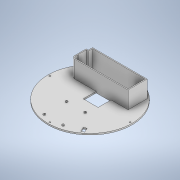
# Autodesk Inventor part: 07_CaseTop
Saved by Autodesk Inventor 2021 (Build 250183000, 183)
## iProperties
Created: 2021-06-07
Part Number: 07_CaseTop
Material: Generisch
Document SubType Name: Modeling
Designer: User
Density: 1 g/cm^3
Appearance: Vorgabe
Author: User
Autodesk Inventor part; units mm, degrees
ref_plane "YZ Plane" through (0, 0, 0) normal (1, 0, 0) x (0, 1, 0)
ref_plane "XZ Plane" through (0, 0, 0) normal (0, 1, 0) x (-1, 0, 0)
ref_plane "XY Plane" through (0, 0, 0) normal (0, 0, 1) x (1, 0, 0)
derived "00_Mastersketch.ipt"
sketch "03_caseTopSketch" plane through (0, 36, 0) normal (0, 1, 0) x (-1, 0, 0)
  line L0 (65.75, -28.4858) -> (65.75, -72.4858) construction
  line L1 (65.75, -72.4858) -> (-71.25, -72.4858) construction
  line L2 (-71.25, -72.4858) -> (-71.25, -28.4858) construction
  line L3 (-71.25, -28.4858) -> (65.75, -28.4858) construction
  line L4 (65.75, -50.4858) -> (-71.25, -50.4858) construction
  arc A0 (65.75, -39.4858) -> (65.75, -28.4858) centre (65.75, -33.9858) ccw construction
  line L5 (65.75, -28.0858) -> (-71.65, -28.0858)
  line L6 (-71.65, -28.0858) -> (-71.65, -72.8858)
  line L7 (-71.65, -72.8858) -> (66.15, -72.8858)
  arc A1 (65.75, -39.8858) -> (67.8854, -39.4858) centre (65.75, -33.9858) ccw
  line L8 (-74.05, -25.6858) -> (65.75, -25.6858)
  arc A2 (74.05, -33.9858) -> (65.75, -25.6858) centre (65.75, -33.9858) ccw
  line L9 (68.55, -75.2858) -> (-74.05, -75.2858)
  line L10 (-74.05, -75.2858) -> (-74.05, -25.6858)
  circle A3 centre (0, 0) radius 110
  circle A4 centre (0, 0) radius 110
  line L11 (74.05, -33.9858) -> (74.05, -63.8858)
  line L12 (74.05, -63.8858) -> (68.55, -63.8858)
  line L13 (67.8854, -39.4858) -> (70.77, -39.4858)
  line L14 (71.65, -39.4858) -> (71.65, -61.4858)
  line L15 (71.65, -61.4858) -> (66.15, -61.4858)
  line L16 (68.55, -63.8858) -> (68.55, -75.2858)
  line L17 (66.15, -72.8858) -> (66.15, -61.4858)
  line L18 (74.05, -39.8858) -> (65.75, -39.8858) construction
  circle A5 centre (0, 0) radius 107.6
  line L19 (-74.05, -75.2858) -> (-75.4525, -76.7117) construction
  line L20 (-24.5, 37) -> (-24.5, 95) construction
  line L21 (24.5, 37) -> (-24.5, 37) construction
  line L22 (-24.5, 95) -> (24.5, 95) construction
  circle A6 centre (-24.5, 37) radius 1.35 construction
  circle A7 centre (-24.5, 37) radius 3 construction
  circle A8 centre (-24.5, 95) radius 1.35 construction
  circle A9 centre (-24.5, 95) radius 3 construction
  line L23 (24.5, 95) -> (24.5, 37) construction
  circle A10 centre (24.5, 37) radius 1.35 construction
  circle A11 centre (24.5, 37) radius 3 construction
  circle A12 centre (24.5, 95) radius 1.4 construction
  circle A13 centre (24.5, 95) radius 3 construction
  line L24 (0, -205.8736) -> (0, 465.2416)
  circle A14 centre (0, 105) radius 5
  line L25 (-29.5, 8.3142) -> (-29.5, -25.6858)
  line L26 (-29.5, -25.6858) -> (9.5, -25.6858)
  line L27 (9.5, -25.6858) -> (9.5, 8.3142)
  line L28 (9.5, 8.3142) -> (-29.5, 8.3142)
  line L29 (67.8854, -39.4858) -> (62.65, -39.4858)
  line L30 (62.65, -39.4858) -> (62.65, -61.4858)
  line L31 (62.65, -61.4858) -> (66.15, -61.4858)
  arc A15 (67.8854, -39.4858) -> (70.77, -37.0858) centre (65.75, -33.9858) ccw construction
  line L32 (70.77, -37.0858) -> (70.77, -39.4858)
  arc A16 (70.77, -37.0858) -> (65.75, -28.0858) centre (65.75, -33.9858) ccw
  line L33 (70.77, -39.4858) -> (71.65, -39.4858)
  point P0 (-29.5, -25.6858)
  point P1 (9.5, -25.6858)
  dimension "d39" = 39
  dimension "d40" = 34
  dimension "d43" = 5
  dimension "d45" = 9
  measures "d39" distance between parallel lines of L27 L25
  measures "d40" distance between parallel lines of L26 L28
  measures "d43" distance between parallel lines of L20 L25
  measures "d45" distance between parallel lines of L14 L30
extrude "Extrusion1" add sketch "03_caseTopSketch" along normal blind 3.6
extrude "Extrusion2" add sketch "03_caseTopSketch" along normal blind 48.6 contours L5 L24 L8 A2 L11 L12 L16 L9 L7 L17 L15 L14 L33 L32 A16 | L5 L6 L7 L24 L9 L10 L8
hole "Bohrung1" at (0, 36, 105) direction (0, 1, 0) diameter 3.8 depth 5 tip angle 118
pattern_circular "Runde Anordnung1" count 4 over 360 about axis through (0, -10, 0) along (0, 1, 0) of "Bohrung1"
sketch "Skizze2" plane through (0, 39.6, 0) normal (0, 1, 0) x (1, 0, 0)
  circle A0 centre (24.5, -37) radius 3 construction
  circle A1 centre (24.5, -37) radius 1.35 construction
  circle A2 centre (24.5, -95) radius 3 construction
  circle A3 centre (24.5, -95) radius 1.35 construction
  circle A4 centre (-24.5, -95) radius 3 construction
  circle A5 centre (-24.5, -95) radius 1.4 construction
  circle A6 centre (-24.5, -37) radius 3 construction
  circle A7 centre (-24.5, -37) radius 1.35 construction
  circle A8 centre (24.5, -37) radius 1.35
  circle A9 centre (24.5, -37) radius 2.9
  circle A10 centre (24.5, -95) radius 1.35
  circle A11 centre (24.5, -95) radius 2.9
  circle A12 centre (-24.5, -95) radius 1.4
  circle A13 centre (-24.5, -95) radius 2.9
  circle A14 centre (-24.5, -37) radius 1.35
  circle A15 centre (-24.5, -37) radius 2.9
  line L0 (67.9237, -81.5229) -> (62.3349, -69.7855)
  line L1 (62.3349, -69.7855) -> (55.1119, -73.2248)
  line L2 (55.1119, -73.2248) -> (60.7007, -84.9621)
  line L3 (60.7007, -84.9621) -> (67.9237, -81.5229)
  line L4 (65.1293, -75.6542) -> (24.5, -95) construction
  line L5 (70.4129, -84.5105) -> (67.9237, -81.5229) construction
  circle A16 centre (0, 0) radius 110 projected
  point P0 (57.9063, -79.0935)
  dimension "d27" = 0.1
  dimension "d34" = 13
  dimension "d35" = 8
  dimension "d36" = 45
  constraints: 12 end point, 8 centre point, 8 coincident, 7 equal radius, 2 midpoint, 1 parallel, 1 perpendicular, 1 point on line, 4 other
  measures "d27" radial gap between concentric circles of A9 A0
  measures "d34" distance between parallel lines of L1 L3
  measures "d35" distance between parallel lines of L2 L0
  measures "d36" distance of L4.start L4.end
extrude "Extrusion5" cut sketch "Skizze2" against normal through all contours A8 | A10 | A12 | A14
extrude "Extrusion6" add sketch "Skizze2" along normal blind 1.6 contours A9 | A11 | A13 | A15
extrude "Extrusion7" cut sketch "03_caseTopSketch" along normal through all contours L33 L14 L15 L31 L30 L29 L13
extrude "Extrusion8" cut sketch "Skizze2" along normal through all both and the other way through all contours L3 L2 L1 L0
extrude "Extrusion9" cut sketch "03_caseTopSketch" along normal through all contours L24 L28 L27 L8 | L8 L25 L28 L24
equation "\"d3\" = TopThickness"
equation "\"TopThickness\" = 3.6"
